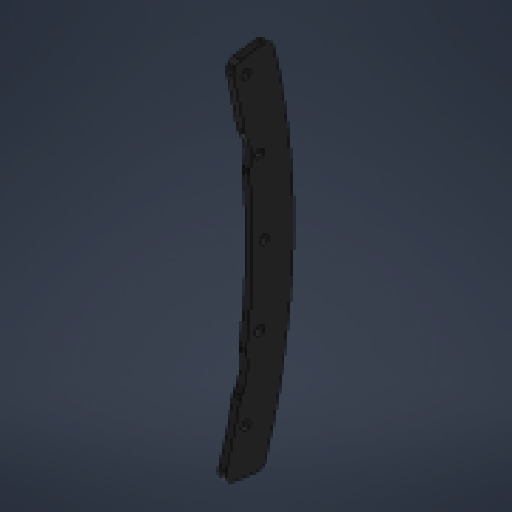
# Autodesk Inventor part: 3DPRINT,HOOD,ALIGNMENT,PLATES
Saved by Autodesk Inventor 2026.1 (Build 301233020, 233B)
## iProperties
Created: 2026-01-30
Part Number: 3DPRINT,HOOD,ALIGNMENT,PLATES
Material: Nylon 6/6
Document SubType Name: Modeling
Designer: Owen L
Density: 1.13 g/cm^3
Appearance: Smooth - Black
Author: Owen L
Autodesk Inventor part; units mm, degrees
ref_plane "YZ Plane" through (0, 0, 0) normal (1, 0, 0) x (0, 1, 0)
ref_plane "XZ Plane" through (0, 0, 0) normal (0, 1, 0) x (-1, 0, 0)
ref_plane "XY Plane" through (0, 0, 0) normal (0, 0, 1) x (1, 0, 0)
sketch "Sketch1" plane through (0, 0, 0) normal (1, 0, 0) x (0, 1, 0)
  arc A0 (-67.3092, -213.4776) -> (57.9334, -216.2104) centre (0, 0) ccw
  arc A1 (-69.6961, -221.0477) -> (59.9878, -223.8775) centre (0, 0) ccw construction
  line L0 (0, 0) -> (-69.6961, -221.0477) construction
  line L1 (0, 0) -> (59.9878, -223.8775) construction
  line L2 (59.9878, -223.8775) -> (57.9334, -216.2104) construction
  line L3 (0, -287.3347) -> (0, 47.8891) construction
  arc A2 (-69.6961, -227.6971) -> (59.9878, -230.4452) centre (0, 0) ccw
  arc A3 (-68.5027, -217.2627) -> (58.9606, -220.0439) centre (0, 0) ccw construction
  arc A4 (-68.5027, -217.2627) -> (-53.1803, -221.5119) centre (0, 0) ccw
  line L4 (-53.1803, -221.5119) -> (0, 0) construction
  arc A5 (-35.1466, -206.5815) -> (27.3518, -207.7573) centre (0, 0) ccw construction
  line L5 (0, 0) -> (27.3518, -207.7573) construction
  line L6 (0, 0) -> (209.55, 0) construction
  circle A6 centre (27.3518, -207.7573) radius 15.5575
  circle A7 centre (-35.1466, -206.5815) radius 15.5575
  line L7 (59.9878, -230.4452) -> (57.9334, -216.2104)
  line L8 (-69.6961, -227.6971) -> (-67.3092, -213.4776)
  point P0 (-26.7758, -226.2272)
  point P1 (0, -227.8063)
  point P2 (26.7758, -226.2272)
  point P3 (53.1803, -221.5119)
  point P4 (35.5128, -221.0024)
  point P5 (22.8969, -222.6633)
  point P6 (-31.2556, -221.6446)
  point P7 (-43.8, -219.5103)
  dimension "d0" = 223.8375
  dimension "d1" = 231.775
  dimension "d2" = 32.5
  dimension "d3" = 15
  dimension "d4" = 238.125
  dimension "d5" = 4
  dimension "d8" = 27
  dimension "d19" = 209.55
  dimension "d20" = 82.5
  dimension "d21" = 62.5094
  dimension "d22" = 31.115
  dimension "d23" = 31.115
  constraints: 16 end point, 13 point on circle, 8 centre point, 8 coincident, 2 point on line, 2 vertical alignment, 1 collinear, 1 equal length, 1 horizontal, 1 midpoint, 5 other
  measures "d0" radius of A0
  measures "d1" radius of A1
  measures "d2" angle of L0 L1
  measures "d3" angle of L3 L1
  measures "d4" radius of A2
  measures "d5" angle of L0 L4
  measures "d19" radius of A5
  measures "d20" angle of L5 L6
  measures "d21" distance of L5.end A5.start
  measures "d22" diameter of A6
  measures "d23" diameter of A7
extrude "Extrusion1" add sketch "Sketch1" along normal blind 2.54 contours A0 A7 A6 L7 A2 L8
hole "Hole1" at (0, -53.1803, -221.5119) at (0, -26.7758, -226.2272) at (0, 0, -227.8063) at (0, 26.7758, -226.2272) at (0, 53.1803, -221.5119) direction (1, 0, 0) diameter 3.2004 end through all clearance for "Flat Head Machine Screw" size "M3" standard "Ansi Metric M Profile"
fillet "Fillet1" radius 3.175 8 edges at (1.27, 57.9334, -216.2104) (1.27, 59.9878, -230.4452) (1.27, 35.5128, -221.0024) (1.27, 22.8969, -222.6633) (1.27, -31.2556, -221.6446) (1.27, -43.8, -219.5103) (1.27, -67.3092, -213.4776) (1.27, -69.6961, -227.6971)
body "Solid1"
